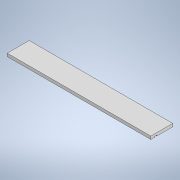
# Autodesk Inventor part: big bourd
Saved by Autodesk Inventor 2021 (Build 250183000, 183)
## iProperties
Created: 2021-07-05
Part Number: big bourd
Material: Generic
Document SubType Name: Modeling
Designer: newic
Density: 1 g/cm^3
Appearance: Default
Author: newic
Autodesk Inventor part; units mm, degrees
ref_plane "YZ Plane" through (0, 0, 0) normal (1, 0, 0) x (0, 1, 0)
ref_plane "XZ Plane" through (0, 0, 0) normal (0, 1, 0) x (-1, 0, 0)
ref_plane "XY Plane" through (0, 0, 0) normal (0, 0, 1) x (1, 0, 0)
sketch "Sketch1" plane through (0, 0, 0) normal (1, 0, 0) x (0, 1, 0)
  line L0 (0, 0) -> (19.05, 0)
  line L1 (19.05, 0) -> (19.05, -139.7)
  line L2 (19.05, -139.7) -> (0, -139.7)
  line L3 (0, -139.7) -> (0, 0)
  dimension "d0" = 19.05
  dimension "d1" = 139.7
  constraints: 8 end point, 2 parallel, 1 horizontal, 1 perpendicular
  measures "d0" distance of L1.end L2.end
  measures "d1" distance of L0.end L1.end
extrude "Extrusion1" add sketch "Sketch1" along normal blind 914.4
sketch "Sketch2" plane through (0, 0, 0) normal (-1, 0, 0) x (0, 0, 1)
  line L0 (0, 19.05) -> (0, 0) projected
  line L1 (0, 9.525) -> (-25.4, 9.525)
  line L2 (-25.4, 9.525) -> (-38.1, 9.525)
  line L3 (0, 0) -> (-139.7, 0) projected
  line L4 (-139.7, 5.08) -> (-5.08, 5.08)
  line L5 (-5.08, 5.08) -> (-5.08, 19.05)
  line L6 (-38.1, 5.08) -> (-38.1, 0)
  line L7 (0, 0) -> (-139.7, 0) projected
  line L8 (-25.4, 5.08) -> (-25.4, 0)
  dimension "d4" = 25.4
  dimension "d5" = 12.7
  dimension "d6" = 5.08
  constraints: 12 end point, 4 point on line, 2 horizontal, 2 perpendicular, 1 midpoint, 1 other
  measures "d4" distance of L1.start L1.end
  measures "d5" distance of L1.end L2.end
  measures "d6" distance between parallel lines of L3 L4
extrude "Extrusion2" cut sketch "Sketch2" against normal through all contours L3 L6 L4 L8
body "Solid1"
